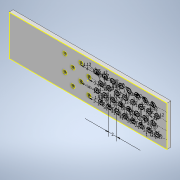
# Autodesk Inventor part: Front Panel
Saved by Autodesk Inventor 2021.4 (Build 254397000, 397)
## iProperties
Created: 2022-05-05
Part Number: Front Panel
Material: Generic
Document SubType Name: Modeling
Designer: LaborAdmin
Density: 1 g/cm^3
Appearance: Default
Author: LaborAdmin
Autodesk Inventor part; units mm, degrees
ref_plane "YZ Plane" through (0, 0, 0) normal (1, 0, 0) x (0, 1, 0)
ref_plane "XZ Plane" through (0, 0, 0) normal (0, 1, 0) x (-1, 0, 0)
ref_plane "XY Plane" through (0, 0, 0) normal (0, 0, 1) x (1, 0, 0)
sketch "Sketch1" plane through (0, 0, 0) normal (0, 0, 1) x (1, 0, 0)
  line L0 (241, -66.5) -> (-241, -66.5)
  line L1 (-241, -66.5) -> (-241, 66.5)
  line L2 (-241, 66.5) -> (241, 66.5)
  line L3 (241, 66.5) -> (241, -66.5)
  line L4 (241, -66.5) -> (-241, 66.5) construction
  line L5 (-241, -66.5) -> (241, 66.5) construction
  line L6 (197, -50) -> (-197, -50)
  line L7 (-197, -50) -> (-197, 50)
  line L8 (-197, 50) -> (197, 50)
  line L9 (197, 50) -> (197, -50)
  line L10 (197, -50) -> (-197, 50) construction
  line L11 (-197, -50) -> (197, 50) construction
  line L12 (17, 50) -> (17, -50) construction
  line L13 (-73, 50) -> (-73, -50) construction
  line L14 (-58, 30) -> (-18, 30) construction
  line L15 (-18, 30) -> (17, 30) construction
  line L16 (-38, 10) -> (-73, 10) construction
  line L17 (-38, 10) -> (2, 10) construction
  line L18 (-58, -10) -> (-18, -10) construction
  line L19 (-18, -10) -> (17, -10) construction
  arc A0 (-61.0692, 33.89) -> (-54.9308, 33.89) centre (-58, 30) ccw
  line L20 (-61.0692, 33.89) -> (-54.9308, 33.89)
  arc A1 (-21.0692, 33.89) -> (-14.9308, 33.89) centre (-18, 30) ccw
  line L21 (-21.0692, 33.89) -> (-14.9308, 33.89)
  arc A2 (-41.0692, 13.89) -> (-34.9308, 13.89) centre (-38, 10) ccw
  arc A3 (-1.0692, 13.89) -> (5.0692, 13.89) centre (2, 10) ccw
  arc A4 (-1.0692, -26.11) -> (5.0692, -26.11) centre (2, -30) ccw
  arc A5 (-41.0692, -26.11) -> (-34.9308, -26.11) centre (-38, -30) ccw
  line L22 (-41.0692, 13.89) -> (-34.9308, 13.89)
  line L23 (-1.0692, 13.89) -> (5.0692, 13.89)
  line L24 (-41.0692, -26.11) -> (-34.9308, -26.11)
  line L25 (-1.0692, -26.11) -> (5.0692, -26.11)
  arc A6 (-61.0692, -6.11) -> (-54.9308, -6.11) centre (-58, -10) ccw
  arc A7 (-21.0692, -6.11) -> (-14.9308, -6.11) centre (-18, -10) ccw
  line L26 (-61.0692, -6.11) -> (-54.9308, -6.11)
  line L27 (-21.0692, -6.11) -> (-14.9308, -6.11)
  point P0 (0, 0)
  dimension "d0" = 133
  dimension "d1" = 482
  dimension "d2" = 100
  dimension "d3" = 394
  dimension "d4" = 180
  dimension "d5" = 90
  dimension "d6" = 20
  dimension "d7" = 15
  dimension "d8" = 35
  dimension "d9" = 20
  dimension "d13" = 20
  dimension "d15" = 15
  dimension "d16" = 20
  dimension "d17" = 15
  dimension "d18" = 35
  dimension "d19" = 20
  dimension "d20" = 35
  dimension "d21" = 20
  dimension "d22" = 20
  dimension "d23" = 15
  dimension "d24" = 20
  dimension "d25" = 9.91
  dimension "d26" = 3.89
  dimension "d27" = 9.91
  dimension "d28" = 3.89
  dimension "d29" = 9.91
  dimension "d30" = 9.91
  dimension "d32" = 9.91
  dimension "d33" = 35
  dimension "d34" = 9.91
  dimension "d35" = 3.89
  dimension "d36" = 3.89
  dimension "d37" = 3.89
  dimension "d38" = 3.89
  dimension "d39" = 9.91
  dimension "d40" = 9.91
  dimension "d41" = 3.89
  dimension "d42" = 3.89
  constraints: 56 end point, 16 point on circle, 10 horizontal, 8 centre point, 8 coincident, 7 perpendicular, 7 point on line, 4 midpoint, 4 parallel
  measures "d0" distance of L0.end L1.end
  measures "d1" distance of L1.end L2.end
  measures "d2" distance of L6.end L7.end
  measures "d3" distance of L7.end L8.end
  measures "d4" distance of L8.end L12.start
  measures "d5" distance of L12.start L13.start
  measures "d6" distance from line of L8 L14.start
  measures "d7" distance from line of L13 L14.start
  measures "d8" distance from line of L12 L14.end
  measures "d9" distance from line of L8 L14.end
  measures "d13" distance from line of L14 L16.start
  measures "d15" distance from line of L12 L17.end
  measures "d16" distance from line of L16 L18.start
  measures "d17" distance from line of L13 L18.start
  measures "d18" distance from line of L12 L18.end
  measures "d19" distance from line of L17 L18.end
  measures "d20" distance from line of L13 L16.start
  measures "d21" distance from line of L15 L17.end
  measures "d22" distance from line of L18 point (-38, -30)
  measures "d23" distance from line of L12 point (2, -30)
  measures "d24" distance from line of L19 point (2, -30)
  measures "d25" diameter of A0
  measures "d26" distance from line of L20 A0.centre
  measures "d27" diameter of A1
  measures "d28" distance from line of L21 A1.centre
  measures "d29" diameter of A2
  measures "d30" diameter of A3
  measures "d32" diameter of A4
  measures "d33" distance from line of L13 point (-38, -30)
  measures "d34" diameter of A5
  measures "d35" distance from line of L22 L16.start
  measures "d36" distance from line of L23 L17.end
  measures "d37" distance from line of L24 point (-38, -30)
  measures "d38" distance from line of L25 point (2, -30)
  measures "d39" diameter of A6
  measures "d40" diameter of A7
  measures "d41" distance from line of L26 A6.centre
  measures "d42" distance from line of L27 L18.end
extrude "Extrusion1" add sketch "Sketch1" along normal blind 10 contours L6 L7 L8 L9
sketch "Sketch2" plane through (0, 0, 10) normal (0, 0, 1) x (1, 0, 0)
  line L0 (197, 50) -> (-197, 50) projected
  line L1 (-197, 50) -> (-197, -50) projected
  line L2 (-197, -50) -> (197, -50) projected
  line L3 (197, -50) -> (197, 50) projected
  line L4 (-21.0692, -6.11) -> (-14.9308, -6.11) projected
  arc A0 (-21.0692, -6.11) -> (-14.9308, -6.11) centre (-18, -10) ccw projected
  line L5 (-61.0692, -6.11) -> (-54.9308, -6.11) projected
  arc A1 (-61.0692, -6.11) -> (-54.9308, -6.11) centre (-58, -10) ccw projected
  line L6 (-41.0692, -26.11) -> (-34.9308, -26.11) projected
  arc A2 (-41.0692, -26.11) -> (-34.9308, -26.11) centre (-38, -30) ccw projected
  line L7 (-1.0692, -26.11) -> (5.0692, -26.11) projected
  arc A3 (-1.0692, -26.11) -> (5.0692, -26.11) centre (2, -30) ccw projected
  line L8 (-1.0692, 13.89) -> (5.0692, 13.89) projected
  arc A4 (-1.0692, 13.89) -> (5.0692, 13.89) centre (2, 10) ccw projected
  line L9 (-41.0692, 13.89) -> (-34.9308, 13.89) projected
  arc A5 (-41.0692, 13.89) -> (-34.9308, 13.89) centre (-38, 10) ccw projected
  line L10 (-21.0692, 33.89) -> (-14.9308, 33.89) projected
  arc A6 (-21.0692, 33.89) -> (-14.9308, 33.89) centre (-18, 30) ccw projected
  line L11 (-61.0692, 33.89) -> (-54.9308, 33.89) projected
  arc A7 (-61.0692, 33.89) -> (-54.9308, 33.89) centre (-58, 30) ccw projected
  point P0 (0, 0)
sketch "Sketch3" plane through (0, 0, 10) normal (0, 0, 1) x (1, 0, 0)
  point P0 (0, 0)
sketch "Sketch4" plane through (0, 0, 10) normal (0, 0, 1) x (1, 0, 0)
  arc A0 (-21.0692, 33.89) -> (-14.9308, 33.89) centre (-18, 30) ccw projected
  line L0 (-18, 30) -> (197, 30) construction
  line L1 (197, -50) -> (197, 50) projected
  arc A1 (-1.0692, 13.89) -> (5.0692, 13.89) centre (2, 10) ccw projected
  line L2 (2, 10) -> (197, 10) construction
  arc A2 (-21.0692, -6.11) -> (-14.9308, -6.11) centre (-18, -10) ccw projected
  line L3 (-18, -10) -> (197, -10) construction
  arc A3 (-1.0692, -26.11) -> (5.0692, -26.11) centre (2, -30) ccw projected
  line L4 (2, -30) -> (197, -30) construction
  line L5 (-197, -50) -> (197, -50) projected
  arc A4 (29.687, 15.1) -> (34.313, 15.1) centre (32, 10) ccw
  arc A5 (49.687, 15.1) -> (54.313, 15.1) centre (52, 10) ccw
  arc A6 (69.687, 15.1) -> (74.313, 15.1) centre (72, 10) ccw
  arc A7 (89.687, 15.1) -> (94.313, 15.1) centre (92, 10) ccw
  arc A8 (109.687, 15.1) -> (114.313, 15.1) centre (112, 10) ccw
  arc A9 (129.687, 15.1) -> (134.313, 15.1) centre (132, 10) ccw
  arc A10 (149.687, 15.1) -> (154.313, 15.1) centre (152, 10) ccw
  arc A11 (169.687, 15.1) -> (174.313, 15.1) centre (172, 10) ccw
  arc A12 (19.687, -4.9) -> (24.313, -4.9) centre (22, -10) ccw
  arc A13 (39.687, -4.9) -> (44.313, -4.9) centre (42, -10) ccw
  arc A14 (59.687, -4.9) -> (64.313, -4.9) centre (62, -10) ccw
  arc A15 (79.687, -4.9) -> (84.313, -4.9) centre (82, -10) ccw
  arc A16 (99.687, -4.9) -> (104.313, -4.9) centre (102, -10) ccw
  arc A17 (119.687, -4.9) -> (124.313, -4.9) centre (122, -10) ccw
  arc A18 (139.687, -4.9) -> (144.313, -4.9) centre (142, -10) ccw
  arc A19 (159.687, -4.9) -> (164.313, -4.9) centre (162, -10) ccw
  arc A20 (19.687, 35.1) -> (24.313, 35.1) centre (22, 30) ccw
  arc A21 (39.687, 35.1) -> (44.313, 35.1) centre (42, 30) ccw
  arc A22 (59.687, 35.1) -> (64.313, 35.1) centre (62, 30) ccw
  arc A23 (79.687, 35.1) -> (84.313, 35.1) centre (82, 30) ccw
  arc A24 (99.687, 35.1) -> (104.313, 35.1) centre (102, 30) ccw
  arc A25 (119.687, 35.1) -> (124.313, 35.1) centre (122, 30) ccw
  arc A26 (139.687, 35.1) -> (144.313, 35.1) centre (142, 30) ccw
  arc A27 (159.687, 35.1) -> (164.313, 35.1) centre (162, 30) ccw
  arc A28 (29.687, -24.9) -> (34.313, -24.9) centre (32, -30) ccw
  arc A29 (49.687, -24.9) -> (54.313, -24.9) centre (52, -30) ccw
  arc A30 (69.687, -24.9) -> (74.313, -24.9) centre (72, -30) ccw
  arc A31 (89.687, -24.9) -> (94.313, -24.9) centre (92, -30) ccw
  arc A32 (109.687, -24.9) -> (114.313, -24.9) centre (112, -30) ccw
  arc A33 (129.687, -24.9) -> (134.313, -24.9) centre (132, -30) ccw
  arc A34 (149.687, -24.9) -> (154.313, -24.9) centre (152, -30) ccw
  arc A35 (169.687, -24.9) -> (174.313, -24.9) centre (172, -30) ccw
  line L6 (159.687, -4.9) -> (164.313, -4.9)
  line L7 (139.687, -4.9) -> (144.313, -4.9)
  line L8 (119.687, -4.9) -> (124.313, -4.9)
  line L9 (99.687, -4.9) -> (104.313, -4.9)
  line L10 (79.687, -4.9) -> (84.313, -4.9)
  line L11 (59.687, -4.9) -> (64.313, -4.9)
  line L12 (19.687, -4.9) -> (24.313, -4.9)
  line L13 (39.687, -4.9) -> (44.313, -4.9)
  line L14 (19.687, 35.1) -> (24.313, 35.1)
  line L15 (39.687, 35.1) -> (44.313, 35.1)
  line L16 (59.687, 35.1) -> (64.313, 35.1)
  line L17 (79.687, 35.1) -> (84.313, 35.1)
  line L18 (99.687, 35.1) -> (104.313, 35.1)
  line L19 (119.687, 35.1) -> (124.313, 35.1)
  line L20 (139.687, 35.1) -> (144.313, 35.1)
  line L21 (159.687, 35.1) -> (164.313, 35.1)
  circle A36 centre (22, 30) radius 8 construction
  circle A37 centre (42, 30) radius 8 construction
  line L22 (29.687, 15.1) -> (34.313, 15.1)
  line L23 (49.687, 15.1) -> (54.313, 15.1)
  line L24 (69.687, 15.1) -> (74.313, 15.1)
  line L25 (89.687, 15.1) -> (94.313, 15.1)
  line L26 (109.687, 15.1) -> (114.313, 15.1)
  line L27 (129.687, 15.1) -> (134.313, 15.1)
  line L28 (149.687, 15.1) -> (154.313, 15.1)
  line L29 (169.687, 15.1) -> (174.313, 15.1)
  line L30 (29.687, -24.9) -> (34.313, -24.9)
  line L31 (49.687, -24.9) -> (54.313, -24.9)
  line L32 (69.687, -24.9) -> (74.313, -24.9)
  line L33 (89.687, -24.9) -> (94.313, -24.9)
  line L34 (109.687, -24.9) -> (114.313, -24.9)
  line L35 (129.687, -24.9) -> (134.313, -24.9)
  line L36 (149.687, -24.9) -> (154.313, -24.9)
  line L37 (169.687, -24.9) -> (174.313, -24.9)
  point P0 (0, 0)
  dimension "d46" = 30
  dimension "d47" = 20
  dimension "d48" = 20
  dimension "d49" = 20
  dimension "d50" = 20
  dimension "d51" = 20
  dimension "d52" = 20
  dimension "d53" = 20
  dimension "d54" = 11.2
  dimension "d55" = 11.2
  dimension "d56" = 11.2
  dimension "d57" = 11.2
  dimension "d58" = 11.2
  dimension "d59" = 11.2
  dimension "d60" = 11.2
  dimension "d61" = 11.2
  dimension "d62" = 40
  dimension "d63" = 20
  dimension "d64" = 20
  dimension "d65" = 20
  dimension "d66" = 20
  dimension "d67" = 20
  dimension "d68" = 20
  dimension "d69" = 20
  dimension "d70" = 11.2
  dimension "d71" = 11.2
  dimension "d72" = 11.2
  dimension "d73" = 11.2
  dimension "d74" = 11.2
  dimension "d75" = 11.2
  dimension "d76" = 11.2
  dimension "d77" = 11.2
  dimension "d78" = 40
  dimension "d79" = 20
  dimension "d80" = 20
  dimension "d81" = 20
  dimension "d82" = 20
  dimension "d83" = 20
  dimension "d84" = 20
  dimension "d85" = 20
  dimension "d86" = 11.2
  dimension "d87" = 11.2
  dimension "d88" = 11.2
  dimension "d89" = 11.2
  dimension "d90" = 11.2
  dimension "d91" = 11.2
  dimension "d92" = 11.2
  dimension "d93" = 11.2
  dimension "d94" = 11.2
  dimension "d95" = 11.2
  dimension "d96" = 11.2
  dimension "d97" = 11.2
  dimension "d98" = 11.2
  dimension "d99" = 11.2
  dimension "d100" = 11.2
  dimension "d101" = 11.2
  dimension "d104" = 10.7
  dimension "d106" = 10.7
  dimension "d107" = 10.7
  dimension "d108" = 10.7
  dimension "d109" = 10.7
  dimension "d110" = 10.7
  dimension "d111" = 10.7
  dimension "d112" = 10.7
  constraints: 64 end point, 64 point on circle, 34 centre point, 34 coincident, 32 horizontal, 4 point on line, 2 vertical, 44 other
  measures "d46" distance of A1.centre point (32, 10)
  measures "d47" distance of point (52, 10) point (32, 10)
  measures "d48" distance of point (72, 10) point (52, 10)
  measures "d49" distance of point (92, 10) point (72, 10)
  measures "d50" distance of point (112, 10) point (92, 10)
  measures "d51" distance of point (132, 10) point (112, 10)
  measures "d52" distance of point (132, 10) point (152, 10)
  measures "d53" distance of point (172, 10) point (152, 10)
  measures "d54" diameter of A4
  measures "d55" diameter of A5
  measures "d56" diameter of A6
  measures "d57" diameter of A7
  measures "d58" diameter of A8
  measures "d59" diameter of A9
  measures "d60" diameter of A10
  measures "d61" diameter of A11
  measures "d62" distance of A2.centre point (22, -10)
  measures "d63" distance of point (22, -10) point (42, -10)
  measures "d64" distance of point (42, -10) point (62, -10)
  measures "d65" distance of point (62, -10) point (82, -10)
  measures "d66" distance of point (82, -10) point (102, -10)
  measures "d67" distance of point (102, -10) point (122, -10)
  measures "d68" distance of point (122, -10) point (142, -10)
  measures "d69" distance of point (142, -10) point (162, -10)
  measures "d70" diameter of A12
  measures "d71" diameter of A13
  measures "d72" diameter of A14
  measures "d73" diameter of A15
  measures "d74" diameter of A16
  measures "d75" diameter of A17
  measures "d76" diameter of A18
  measures "d77" diameter of A19
  measures "d78" distance of point (22, 30) A0.centre
  measures "d79" distance of point (22, 30) point (42, 30)
  measures "d80" distance of point (42, 30) point (62, 30)
  measures "d81" distance of point (62, 30) point (82, 30)
  measures "d82" distance of point (82, 30) point (102, 30)
  measures "d83" distance of point (102, 30) point (122, 30)
  measures "d84" distance of point (122, 30) point (142, 30)
  measures "d85" distance of point (142, 30) point (162, 30)
  measures "d86" diameter of A20
  measures "d87" diameter of A21
  measures "d88" diameter of A22
  measures "d89" diameter of A23
  measures "d90" diameter of A24
  measures "d91" diameter of A25
  measures "d92" diameter of A26
  measures "d93" diameter of A27
  measures "d94" diameter of A28
  measures "d95" diameter of A29
  measures "d96" diameter of A30
  measures "d97" diameter of A31
  measures "d98" diameter of A32
  measures "d99" diameter of A33
  measures "d100" diameter of A34
  measures "d101" diameter of A35
body "Solid1"
